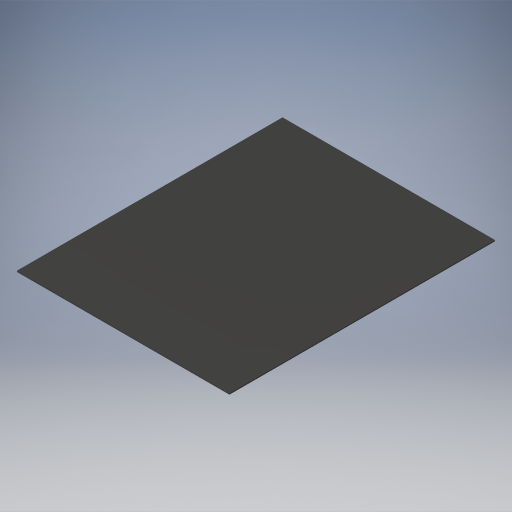
# Autodesk Inventor part: Gummi Matte DRW
Saved by Autodesk Inventor 2023.2 (Build 272271000, 271)
## iProperties
Created: 2023-02-05
Part Number: Gummi Matte DRW
Material: Gummi
Document SubType Name: Modeling
Designer: Raoul Messerli
Density: 0.93 g/cm^3
Appearance: Gummi - Schwarz
Author: Raoul Messerli
Autodesk Inventor part; units mm, degrees
ref_plane "YZ Plane" through (0, 0, 0) normal (1, 0, 0) x (0, 1, 0)
ref_plane "XZ Plane" through (0, 0, 0) normal (0, 1, 0) x (-1, 0, 0)
ref_plane "XY Plane" through (0, 0, 0) normal (0, 0, 1) x (1, 0, 0)
sketch "Skizze1" plane through (0, 0, 0) normal (0, 0, 1) x (1, 0, 0)
  line L0 (0, 0) -> (720, 0)
  line L1 (720, 0) -> (720, 900)
  line L2 (720, 900) -> (0, 900)
  line L3 (0, 900) -> (0, 0)
  dimension "d0" = 900
  dimension "d1" = 720
  constraints: 8 end point, 2 parallel, 1 horizontal, 1 perpendicular
  measures "d0" distance of L0.end L1.end
  measures "d1" distance of L1.end L2.end
extrude "Extrusion1" add sketch "Skizze1" along normal blind 3
